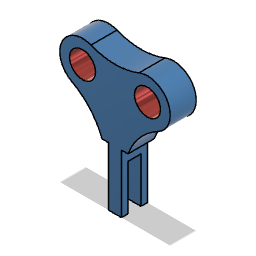
3d12 v1 (Autodesk Fusion 360 design; units mm, degrees)
Autodesk Fusion 360 part; units mm, degrees
sketch "Sketch1" plane through (0, 0, 0) normal (0, 0, 1) x (1, 0, 0)
  circle A0 centre (1.7794, 87) radius 10
  circle A1 centre (51.7794, 87) radius 10
  line L0 (21.7794, 0) -> (31.7794, 0)
  line L1 (31.7794, 0) -> (31.7794, 45)
  line L2 (21.7794, 45) -> (21.7794, 0)
  line L3 (31.7794, 45) -> (36.7794, 45)
  line L4 (21.7794, 45) -> (16.7794, 45)
  arc A2 (60.0311, 71.5676) -> (36.7794, 45) centre (83.6075, 27.4751) ccw
  arc A3 (16.7794, 45) -> (-6.4724, 71.5676) centre (-30.0488, 27.4751) ccw
  arc A4 (8.2609, 103.2555) -> (45.2979, 103.2555) centre (26.7794, 149.6997) ccw
  arc A5 (8.2609, 103.2555) -> (-6.4724, 71.5676) centre (1.7794, 87) ccw
  arc A6 (60.0311, 71.5676) -> (45.2979, 103.2555) centre (51.7794, 87) ccw
  dimension "d1" = 20
  dimension "d2" = 20
  dimension "d3" = 35
  dimension "d4" = 35
  dimension "d5" = 50
  dimension "d6" = 87
  dimension "d7" = 87
  dimension "d8" = 100
  dimension "d9" = 10
  dimension "d10" = 45
  dimension "d11" = 20
  dimension "d12" = 5
  dimension "d13" = 5
  dimension "d14" = 50
  dimension "d15" = 42
  dimension "d16" = 50
  dimension "d17" = 45
  dimension "d18" = 113.6563
  dimension "d19" = 21.7794
  constraint concentric A0 A5
  constraint concentric A1 A6
  constraint tangent A4 A6
  constraint tangent A4 A5
  constraint horizontal L0
  constraint vertical L1
  constraint vertical L2
  constraint perpendicular L1 L3
  constraint perpendicular L2 L4
  constraint tangent A2 A6
  constraint tangent A3 A5
  measures "d1" diameter of A0
  measures "d2" diameter of A1
  measures "d3" diameter of A5
  measures "d4" diameter of A6
  measures "d5" horizontal distance of A0.centre A1.centre
  measures "d6" vertical distance of origin A0.centre
  measures "d7" vertical distance of origin A1.centre
  measures "d8" diameter of A4
  measures "d9" distance of L0.start L0.end
  measures "d10" distance of L0.start L2.start
  measures "d11" horizontal distance of A0.centre L2.start
  measures "d12" distance of L1.end L3.end
  measures "d13" distance of L2.start L4.end
  measures "d14" radius of A2
  measures "d15" vertical distance of A1.centre L1.end
  measures "d16" radius of A3
  measures "d17" distance of L0.end L1.end
  measures "d18" distance of A2.centre A3.centre
  measures "d19" distance of origin L2
extrude "Extrude1" add sketch "Sketch1" along normal mid plane 20
sketch "Sketch2" plane through (31.7794, 0, 0) normal (1, 0, 0) x (0, 0, -1)
  line L0 (10, 45) -> (-10, 45)
  line L1 (-10, 45) -> (-10, 0)
  line L2 (-10, 0) -> (10, 0)
  line L3 (10, 0) -> (10, 45)
  line L4 (-5, 0) -> (-5, 35)
  line L5 (-5, 35) -> (5, 35)
  line L6 (5, 35) -> (5, 0)
  dimension "d22" = 10
  dimension "d23" = 5
  dimension "d24" = 35
  constraint coincident L2 L4.start
  constraint perpendicular L2 L4
  constraint perpendicular L4 L5
  constraint coincident L2 L6.end
  constraint perpendicular L5 L6
  measures "d22" distance of L4.end L5.end
  measures "d23" distance of L3 L6
  measures "d24" distance of L5.end L6.end
extrude "Extrude2" cut sketch "Sketch2" against normal blind 10 contours L2 L4 L5 L6
